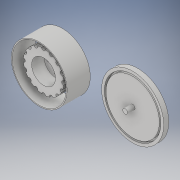
# Autodesk Inventor part: Wheel
Saved by Autodesk Inventor 2017 SP1 (Build 210196100, 196)
## iProperties
Created: 2017-02-11
Part Number: Wheel
Material: Generic
Document SubType Name: Modeling
Designer: Me
Density: 1 g/cm^3
Appearance: Default
Author: Me
Autodesk Inventor part; units mm, degrees
ref_plane "YZ Plane" through (0, 0, 0) normal (1, 0, 0) x (0, 1, 0)
ref_plane "XZ Plane" through (0, 0, 0) normal (0, 1, 0) x (-1, 0, 0)
ref_plane "XY Plane" through (0, 0, 0) normal (0, 0, 1) x (1, 0, 0)
sketch "Sketch1" plane through (0, 0, 0) normal (0, 0, 1) x (1, 0, 0)
  circle A0 centre (0, 0) radius 9.5
  circle A1 centre (0, 6.35) radius 1.425
  circle A2 centre (6.35, 0) radius 1.425
  circle A3 centre (0, -6.35) radius 1.425
  circle A4 centre (-6.35, 0) radius 1.425
  circle A5 centre (0, 0) radius 2
  dimension "d0" = 19
  dimension "d1" = 2.85
  dimension "d2" = 2.85
  dimension "d3" = 2.85
  dimension "d4" = 2.85
  dimension "d5" = 4
  dimension "d6" = 6.35
  dimension "d7" = 6.35
  dimension "d8" = 6.35
  dimension "d9" = 6.35
  constraints: 6 centre point, 2 coincident, 2 horizontal alignment, 2 vertical alignment
  measures "d0" diameter of A0
  measures "d1" diameter of A1
  measures "d2" diameter of A2
  measures "d3" diameter of A3
  measures "d4" diameter of A4
  measures "d5" diameter of A5
  measures "d6" distance of A3.centre point (0, 0)
  measures "d7" distance of A2.centre point (0, 0)
  measures "d8" distance of A1.centre point (0, 0)
  measures "d9" distance of point (0, 0) A4.centre
extrude "Hub Mount" add sketch "Sketch1" along normal blind 5
sketch "Sketch2" plane through (0, 0, 0) normal (0, 0, -1) x (-1, 0, 0)
  circle A0 centre (0, 0) radius 9.5
  circle A1 centre (0, 0) radius 16
  dimension "d12" = 19
  dimension "d13" = 32
  constraints: 2 centre point, 2 coincident
  measures "d12" diameter of A0
  measures "d13" diameter of A1
extrude "Tire Mount" add sketch "Sketch2" against normal blind 15
sketch "Sketch4" plane through (0, 0, 15) normal (0, 0, 1) x (1, 0, 0)
  circle A0 centre (0, 16) radius 1.5
  circle A1 centre (0, 0) radius 16 projected
  circle A2 centre (-16, 0) radius 1.5
  circle A3 centre (0, -16) radius 1.5
  circle A4 centre (16, 0) radius 1.5
  circle A5 centre (0, 0) radius 16 projected
  line L0 (-16, 0) -> (16, 0)
  circle A6 centre (11.3137, 11.3137) radius 1.5
  line L1 (11.3137, 11.3137) -> (0, 0)
  line L2 (0, 0) -> (6.1229, 14.7821)
  line L3 (0, 0) -> (14.7821, 6.1229)
  line L4 (0, 0) -> (14.7821, -6.1229)
  line L5 (0, 0) -> (11.3137, -11.3137)
  line L6 (0, 0) -> (6.1229, -14.7821)
  line L7 (0, 0) -> (-6.1229, -14.7821)
  line L8 (0, 0) -> (-11.3137, -11.3137)
  line L9 (0, 0) -> (-14.7821, -6.1229)
  line L10 (0, 16) -> (0, -16)
  line L11 (0, 0) -> (-6.1229, 14.7821)
  line L12 (0, 0) -> (-11.3137, 11.3137)
  line L13 (0, 0) -> (-14.7821, 6.1229)
  circle A7 centre (6.1229, 14.7821) radius 1.5
  circle A8 centre (14.7821, 6.1229) radius 1.5
  circle A9 centre (14.7821, -6.1229) radius 1.5
  circle A10 centre (11.3137, -11.3137) radius 1.5
  circle A11 centre (6.1229, -14.7821) radius 1.5
  circle A12 centre (-6.1229, -14.7821) radius 1.5
  circle A13 centre (-11.3137, -11.3137) radius 1.5
  circle A14 centre (-14.7821, -6.1229) radius 1.5
  circle A15 centre (-14.7821, 6.1229) radius 1.5
  circle A16 centre (-11.3137, 11.3137) radius 1.5
  circle A17 centre (-6.1229, 14.7821) radius 1.5
  dimension "d21" = 3
  dimension "d22" = 3
  dimension "d23" = 3
  dimension "d24" = 3
  dimension "d29" = 3
  dimension "d30" = 22.5
  dimension "d31" = 22.5
  dimension "d32" = 22.5
  dimension "d33" = 22.5
  dimension "d34" = 22.5
  dimension "d35" = 22.5
  dimension "d36" = 22.5
  dimension "d37" = 22.5
  dimension "d38" = 22.5
  dimension "d39" = 22.5
  dimension "d40" = 22.5
  dimension "d41" = 22.5
  dimension "d42" = 3
  dimension "d43" = 3
  dimension "d44" = 3
  dimension "d45" = 3
  dimension "d46" = 3
  dimension "d47" = 3
  dimension "d48" = 3
  dimension "d49" = 3
  dimension "d50" = 3
  dimension "d51" = 3
  dimension "d52" = 3
  constraints: 28 end point, 16 centre point, 11 coincident, 2 horizontal alignment, 2 vertical alignment, 1 horizontal, 1 vertical, 30 other
  measures "d21" diameter of A2
  measures "d22" diameter of A3
  measures "d23" diameter of A4
  measures "d24" diameter of A0
  measures "d29" diameter of A6
  measures "d30" angle of L0 L3
  measures "d31" angle of L3 L1
  measures "d32" angle of L1 L2
  measures "d33" angle of L0 L4
  measures "d34" angle of L4 L5
  measures "d35" angle of L5 L6
  measures "d36" angle of L10 L7
  measures "d37" angle of L7 L8
  measures "d38" angle of L9 L8
  measures "d39" angle of L10 L11
  measures "d40" angle of L11 L12
  measures "d41" angle of L12 L13
  measures "d42" diameter of A9
  measures "d43" diameter of A10
  measures "d44" diameter of A11
  measures "d45" diameter of A12
  measures "d46" diameter of A13
  measures "d47" diameter of A14
  measures "d48" diameter of A15
  measures "d49" diameter of A16
  measures "d50" diameter of A17
  measures "d51" diameter of A7
  measures "d52" diameter of A8
extrude "Tire Grip Extrusion" cut sketch "Sketch4" against normal through all contours A0 A1 | A1 L10 A0 | A0 L10 A1 | A17 L11 A1 | A1 A17 | A7 A1 | A1 L2 A7 | L11 A17 A1 | A1 A7 L2 | L0 A1 A2 | A2 A1 L0 | L0 A1 A4 | A4 A1 L0 | L1 A1 A6 | A6 A1 L1 | A8 A1 L3 | L3 A1 A8 | A9 A1 L4 | L4 A1 A9 | A10 A1 L5 | L5 A1 A10 | A11 A1 L6 | L6 A1 A11 | A12 A1 L7 | L7 A1 A12 | A13 A1 L8 | L8 A1 A13 | A14 A1 L9 | L9 A1 A14 | L10 A1 A3 | A3 A1 L10 | A16 A1 L12 | L12 A1 A16 | A15 A1 L13 | L13 A1 A15 | A1 A16 | A1 A2 | A4 A1 | A6 A1 | A1 A8 | A1 A9 | A1 A10 | A1 A11 | A1 A12 | A1 A13 | A1 A14 | A3 A1 | A1 A15
sketch "Sketch5" plane through (0, 0, 0) normal (0, 0, -1) x (-1, 0, 0)
  circle A0 centre (0, 0) radius 21.5
  circle A1 centre (0, 0) radius 22.25
  dimension "d55" = 43
  dimension "d56" = 44.5
  constraints: 2 centre point, 2 coincident
  measures "d55" diameter of A0
  measures "d56" diameter of A1
extrude "Tire Mold Shell" add sketch "Sketch5" against normal blind 18.5
sketch "Sketch6" plane through (0, 0, 0) normal (0, 0, -1) x (-1, 0, 0)
  circle A0 centre (-60, 0) radius 24.75
  point P0 (0, 0)
  dimension "d59" = 49.5
  dimension "d60" = 60
  constraints: 1 centre point, 1 horizontal alignment
  measures "d59" diameter of A0
  measures "d60" distance of point (0, 0) A0.centre
extrude "Tire Mold Base" add sketch "Sketch6" against normal blind 4
sketch "Sketch7" plane through (60, 0, 4) normal (0, 0, 1) x (1, 0, 0)
  circle A0 centre (0, 0) radius 22.5
  circle A1 centre (0, 0) radius 21.25
  point P0 (-60, 0)
  dimension "d65" = 42.5
  dimension "d66" = 45
  dimension "d67" = 60
  constraints: 2 centre point, 1 coincident, 1 horizontal alignment
  measures "d65" diameter of A1
  measures "d66" diameter of A0
  measures "d67" distance of A0.centre point (-60, 0)
extrude "Inset into base for shell" cut sketch "Sketch7" against normal blind 2.5
sketch "Sketch8" plane through (60, 0, 4) normal (0, 0, 1) x (1, 0, 0)
  circle A0 centre (0, 0) radius 1.9
  point P0 (-60, 0)
  dimension "d70" = 3.8
  dimension "d71" = 60
  constraints: 1 centre point, 1 horizontal alignment
  measures "d70" diameter of A0
  measures "d71" distance of A0.centre point (-60, 0)
extrude "Extrusion7" add sketch "Sketch8" along normal blind 6
equation "\"d2\" = d1"
equation "\"d3\" = d1"
equation "\"d4\" = d1"
equation "\"d7\" = d6"
equation "\"d8\" = d6"
equation "\"d9\" = d7"
equation "\"d22\" = d21"
equation "\"d23\" = d21"
equation "\"d24\" = d21"
equation "\"d29\" = d24"
equation "\"d31\" = d30"
equation "\"d32\" = d30"
equation "\"d33\" = d30"
equation "\"d34\" = d33"
equation "\"d35\" = d34"
equation "\"d36\" = d30"
equation "\"d37\" = d30"
equation "\"d38\" = d30"
equation "\"d39\" = d30"
equation "\"d40\" = d30"
equation "\"d41\" = d30"
equation "\"d42\" = d21"
equation "\"d43\" = d21"
equation "\"d44\" = d21"
equation "\"d45\" = d21"
equation "\"d46\" = d21"
equation "\"d47\" = d21"
equation "\"d48\" = d21"
equation "\"d49\" = d21"
equation "\"d50\" = d21"
equation "\"d51\" = d21"
equation "\"d52\" = d21"
body "Solid1"
